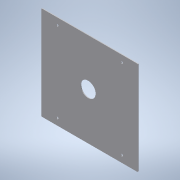
# Autodesk Inventor part: Standard
Saved by Autodesk Inventor 2020.3 (Build 243373000, 373)
## iProperties
RuleStatus: InUse
AfterDocSave0: file://Part Number Cleaner
Created: 2022-04-12
Material: Generic
Catalog Web Link: https://www.janelia.org/
Vendor: HHMI: JRC - jET
Document SubType Name: Modeling
Designer: solomone
Density: 1 g/cm^3
Appearance: Default
DESIGN DEPARTMENT: HHMI: JRC - jET
ALTERED ITEM PART NUMBER: N/A
ALTERED ITEM VENDOR: N/A
ALTERED ITEM DESCRIPTION: N/A
Title: Standard
Author: solomone
Revision Number: 0
Autodesk Inventor part; units mm, degrees
ref_plane "YZ Plane" through (0, 0, 0) normal (1, 0, 0) x (0, 1, 0)
ref_plane "XZ Plane" through (0, 0, 0) normal (0, 1, 0) x (-1, 0, 0)
ref_plane "XY Plane" through (0, 0, 0) normal (0, 0, 1) x (1, 0, 0)
sketch "Sketch1" plane through (0, 0, 0) normal (0, 0, 1) x (1, 0, 0)
  line L0 (203.2, 196.85) -> (-203.2, 196.85)
  line L1 (-203.2, 196.85) -> (-203.2, -196.85)
  line L2 (-203.2, -196.85) -> (203.2, -196.85)
  line L3 (203.2, -196.85) -> (203.2, 196.85)
  point P0 (0, 0)
  dimension "d0" = 393.7
  dimension "d1" = 406.4
  dimension "d2" = 203.2
  dimension "d3" = 196.85
  constraints: 8 end point, 2 parallel, 1 horizontal, 1 perpendicular
  measures "d0" distance of L2.end L0.start
  measures "d1" distance of L0.start L0.end
  measures "d2" distance from line of point (0, 0) L3
  measures "d3" distance from line of point (0, 0) L0
extrude "Extrusion1" add sketch "Sketch1" along normal mid plane 3.175
sketch "Sketch2" plane through (0, 0, 1.5875) normal (0, 0, 1) x (1, 0, 0)
  circle A0 centre (-6.35, 0) radius 31.75
  point P0 (0, 0)
  dimension "d6" = 63.5
  dimension "d20" = 6.35
  constraints: 1 centre point, 1 horizontal alignment
  measures "d6" diameter of A0
  measures "d20" distance of A0.centre point (0, 0)
extrude "Extrusion2" cut sketch "Sketch2" against normal through all
fillet "Fillet1" radius 3.175 4 edges at (203.2, -196.85, 0) (-203.2, -196.85, 0) (-203.2, 196.85, 0) (203.2, 196.85, 0)
sketch "Sketch3" plane through (0, 0, 1.5875) normal (0, 0, 1) x (1, 0, 0)
  line L0 (138.5, 173.4) -> (131.9, 173.4)
  line L1 (131.9, 173.4) -> (131.9, 163.8)
  line L2 (131.9, 163.8) -> (138.5, 163.8)
  line L3 (138.5, 163.8) -> (138.5, 173.4)
  line L4 (135.2, 173.4) -> (135.2, 163.8) construction
  line L5 (203.2, -193.675) -> (203.2, 193.675) projected
  line L6 (200.025, 196.85) -> (-200.025, 196.85) projected
  line L7 (138.5, 168.6) -> (131.9, 168.6) construction
  point P0 (0, 0)
  dimension "d11" = 6.6
  dimension "d12" = 68
  dimension "d14" = 9.6
  dimension "d18" = 28.25
  constraints: 12 end point, 4 midpoint, 2 parallel, 1 horizontal, 1 perpendicular
  measures "d11" distance of L1.end L2.end
  measures "d12" distance between parallel lines of L5 L4
  measures "d14" distance of L0.end L1.end
  measures "d18" distance between parallel lines of L6 L7
extrude "Extrusion3" cut sketch "Sketch3" against normal through all
fillet "Fillet2" radius 3.3 4 edges at (138.5, 173.4, 0) (131.9, 173.4, 0) (138.5, 163.8, 0) (131.9, 163.8, 0)
mirror "Mirror1" about plane through (0, 0, 0) normal (0, 1, 0) of "Extrusion3", "Fillet2"
mirror "Mirror2" about plane through (0, 0, 0) normal (1, 0, 0) of "Extrusion3", "Fillet2", "Mirror1"
equation "\"d2\" = 0.5 * d1"
equation "\"d3\" = 0.5 * d0"
body "Solid1"
